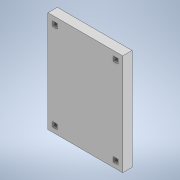
# Autodesk Inventor part: pièce_mobile_station
Saved by Autodesk Inventor 2020.2 (Build 242310000, 310)
## iProperties
Created: 2020-02-25
Part Number: pièce_mobile_station
Material: Générique
Document SubType Name: Modeling
Designer: anton
Density: 1 g/cm^3
Appearance: Par défaut
Author: anton
Autodesk Inventor part; units mm, degrees
ref_plane "YZ Plane" through (0, 0, 0) normal (1, 0, 0) x (0, 1, 0)
ref_plane "XZ Plane" through (0, 0, 0) normal (0, 1, 0) x (-1, 0, 0)
ref_plane "XY Plane" through (0, 0, 0) normal (0, 0, 1) x (1, 0, 0)
sketch "Esquisse1" plane through (0, 0, 0) normal (0, 0, 1) x (1, 0, 0)
  line L0 (-21.137, 18.1163) -> (26.863, 18.1163)
  line L1 (26.863, 18.1163) -> (26.863, -46.8837)
  line L2 (26.863, -46.8837) -> (-21.137, -46.8837)
  line L3 (-21.137, -46.8837) -> (-21.137, 18.1163)
  point P0 (0, 0)
  dimension "d0" = 48
  dimension "d1" = 65
  constraints: 8 end point, 2 parallel, 1 horizontal, 1 perpendicular
  measures "d0" distance of L0.start L0.end
  measures "d1" distance of L2.end L0.start
extrude "Extrusion1" add sketch "Esquisse1" along normal blind 6
sketch "Esquisse2" plane through (0, 0, 6) normal (0, 0, 1) x (1, 0, 0)
  line L0 (-18.137, -40.8837) -> (-15.137, -40.8837)
  line L1 (-15.137, -40.8837) -> (-15.137, -43.8837)
  line L2 (-15.137, -43.8837) -> (-18.137, -43.8837)
  line L3 (-18.137, -43.8837) -> (-18.137, -40.8837)
  line L4 (20.863, -40.8837) -> (23.863, -40.8837)
  line L5 (23.863, -40.8837) -> (23.863, -43.8837)
  line L6 (23.863, -43.8837) -> (20.863, -43.8837)
  line L7 (20.863, -43.8837) -> (20.863, -40.8837)
  line L8 (23.863, 12.1163) -> (20.863, 12.1163)
  line L9 (20.863, 12.1163) -> (20.863, 15.1163)
  line L10 (20.863, 15.1163) -> (23.863, 15.1163)
  line L11 (23.863, 15.1163) -> (23.863, 12.1163)
  line L12 (-15.137, 12.1163) -> (-18.137, 12.1163)
  line L13 (-18.137, 12.1163) -> (-18.137, 15.1163)
  line L14 (-18.137, 15.1163) -> (-15.137, 15.1163)
  line L15 (-15.137, 15.1163) -> (-15.137, 12.1163)
  line L16 (26.863, 18.1163) -> (-21.137, 18.1163) projected
  line L17 (-21.137, 18.1163) -> (-21.137, -46.8837) projected
  line L18 (26.863, -46.8837) -> (26.863, 18.1163) projected
  line L19 (-21.137, -46.8837) -> (26.863, -46.8837) projected
  point P0 (0, 0)
  dimension "d4" = 3
  dimension "d5" = 3
  dimension "d6" = 3
  dimension "d7" = 3
  dimension "d8" = 3
  dimension "d9" = 3
  dimension "d10" = 3
  dimension "d11" = 3
  dimension "d12" = 3
  dimension "d13" = 3
  dimension "d14" = 3
  dimension "d15" = 3
  dimension "d16" = 3
  dimension "d17" = 3
  dimension "d18" = 3
  constraints: 32 end point, 8 parallel, 4 horizontal, 4 perpendicular, 1 point on line
  measures "d4" distance between parallel lines of L16 L14
  measures "d5" distance between parallel lines of L17 L13
  measures "d6" distance of L13.end L14.end
  measures "d7" distance of L12.end L13.end
  measures "d8" distance of L9.end L10.end
  measures "d9" distance of L10.end L8.start
  measures "d10" distance between parallel lines of L11 L18
  measures "d11" distance between parallel lines of L19 L2
  measures "d12" distance between parallel lines of L17 L3
  measures "d13" distance of L2.end L0.start
  measures "d14" distance of L0.start L0.end
  measures "d15" distance of L4.end L5.end
  measures "d16" distance of L4.start L4.end
  measures "d17" distance between parallel lines of L19 L6
  measures "d18" distance between parallel lines of L18 L5
extrude "Extrusion2" cut sketch "Esquisse2" against normal blind 2 contours L0 L1 L2 L3 | L4 L5 L6 L7 | L8 L9 L10 L11 | L12 L13 L14 L15
sketch "Esquisse4" plane through (0, 0, 0) normal (0, 0, -1) x (-1, 0, 0)
  line L0 (-24.863, -1.8837) -> (19.137, -1.8837)
  line L1 (19.137, -1.8837) -> (19.137, -11.8837)
  line L2 (19.137, -11.8837) -> (-24.863, -11.8837)
  line L3 (-24.863, -11.8837) -> (-24.863, -1.8837)
  line L4 (-24.863, -16.8837) -> (19.137, -16.8837)
  line L5 (19.137, -16.8837) -> (19.137, -26.8837)
  line L6 (19.137, -26.8837) -> (-24.863, -26.8837)
  line L7 (-24.863, -26.8837) -> (-24.863, -16.8837)
  line L8 (-24.863, -31.8837) -> (19.137, -31.8837)
  line L9 (19.137, -31.8837) -> (19.137, -41.8837)
  line L10 (19.137, -41.8837) -> (-24.863, -41.8837)
  line L11 (-24.863, -41.8837) -> (-24.863, -31.8837)
  line L12 (-26.863, -46.8837) -> (-26.863, 18.1163) projected
  line L13 (21.137, 18.1163) -> (21.137, -46.8837) projected
  line L14 (-24.863, 13.1163) -> (19.137, 13.1163)
  line L15 (19.137, 13.1163) -> (19.137, 3.1163)
  line L16 (19.137, 3.1163) -> (-24.863, 3.1163)
  line L17 (-24.863, 3.1163) -> (-24.863, 13.1163)
  point P0 (0, 0)
  point P1 (-20.863, 12.1163)
  dimension "d39" = 10
  dimension "d40" = 5
  dimension "d41" = 10
  dimension "d42" = 5
  dimension "d43" = 10
  dimension "d44" = 44
  dimension "d45" = 2
  dimension "d46" = 44
  dimension "d47" = 2
  dimension "d48" = 44
  dimension "d49" = 2
  dimension "d52" = 5
  dimension "d53" = 10
  dimension "d54" = 2
  dimension "d57" = 44
  constraints: 32 end point, 8 parallel, 4 horizontal, 4 perpendicular
  measures "d39" distance of L0.end L1.end
  measures "d40" distance between parallel lines of L2 L4
  measures "d41" distance of L4.end L5.end
  measures "d42" distance between parallel lines of L6 L8
  measures "d43" distance between parallel lines of L8 L10
  measures "d44" distance of L9.end L10.end
  measures "d45" distance between parallel lines of L12 L11
  measures "d46" distance of L5.end L6.end
  measures "d47" distance between parallel lines of L13 L5
  measures "d48" distance of L0.start L0.end
  measures "d49" distance between parallel lines of L13 L1
  measures "d52" distance between parallel lines of L0 L16
  measures "d53" distance between parallel lines of L16 L14
  measures "d54" distance between parallel lines of L13 L15
  measures "d57" distance of L14.start L14.end
extrude "Extrusion4" cut sketch "Esquisse4" against normal blind 1
